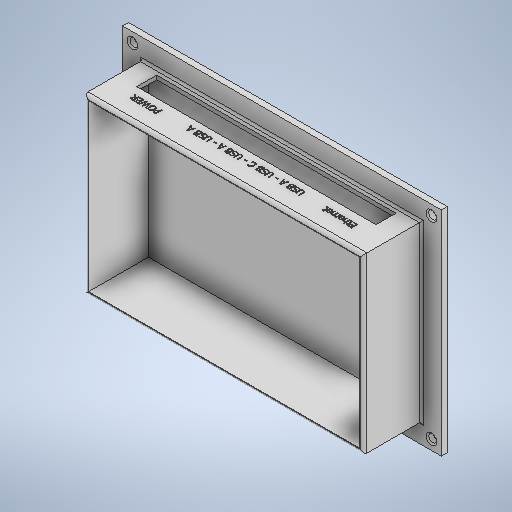
# Autodesk Inventor part: DS Holder
Saved by Autodesk Inventor 2025.1 (Build 291241000, 241)
## iProperties
Created: 2024-09-14
Part Number: DS Holder
Material: Generic
Document SubType Name: Modeling
Designer: ishaa
Density: 1 g/cm^3
Appearance: Default
Author: ishaa
## iProperties of the stored document DS Holder_3DPrint.ipt
Created: 2024-09-15
Part Number: DS Holder_3DPrint
Material: Generic
Document SubType Name: Modeling
Designer: ishaa
Density: 1 g/cm^3
Appearance: Default
Author: ishaa
Autodesk Inventor part; units mm, degrees
ref_plane "YZ Plane" through (0, 0, 0) normal (1, 0, 0) x (0, 1, 0)
ref_plane "XZ Plane" through (0, 0, 0) normal (0, 1, 0) x (-1, 0, 0)
ref_plane "XY Plane" through (0, 0, 0) normal (0, 0, 1) x (1, 0, 0)
sketch "Sketch1" plane through (0, 0, 0) normal (0, 0, 1) x (1, 0, 0)
  line L0 (-70, -43.5) -> (70, -43.5)
  line L1 (70, -43.5) -> (70, 43.5)
  line L2 (70, 43.5) -> (-70, 43.5)
  line L3 (-70, 43.5) -> (-70, -43.5)
  line L4 (-70, -43.5) -> (70, 43.5) construction
  line L5 (70, -43.5) -> (-70, 43.5) construction
  point P0 (0, 0)
  dimension "d0" = 140
  dimension "d1" = 87
  constraints: 12 end point, 2 midpoint, 2 parallel, 1 horizontal, 1 perpendicular
  measures "d0" distance of L2.end L1.end
  measures "d1" distance of L1.end L0.end
extrude "Extrusion1" add sketch "Sketch1" along normal blind 2
sketch "Sketch2" plane through (0, 0, 2) normal (0, 0, 1) x (1, 0, 0)
  line L0 (70, -43.5) -> (70, 43.5) projected
  line L1 (70, 43.5) -> (-70, 43.5) projected
  line L2 (-70, 43.5) -> (-70, -43.5) projected
  line L3 (-70, -43.5) -> (70, -43.5) projected
  line L4 (-68, 41.5) -> (68, 41.5)
  line L5 (68, 41.5) -> (68, -41.5)
  line L6 (68, -41.5) -> (-68, -41.5)
  line L7 (-68, -41.5) -> (-68, 41.5)
  point P0 (0, 0)
  dimension "d4" = 2
  constraints: 8 end point, 3 other
  measures "d4" distance between parallel lines of L1 L4
extrude "Extrusion2" add sketch "Sketch2" along normal blind 30
sketch "Sketch3" plane through (0, 0, 0) normal (0, 0, -1) x (-1, 0, 0)
  line L0 (-70, -43.5) -> (-70, 43.5) projected
  line L1 (70, -43.5) -> (-70, -43.5) projected
  line L2 (70, 43.5) -> (70, -43.5) projected
  line L3 (-70, 43.5) -> (70, 43.5) projected
  line L4 (80, -53.5) -> (-80, -53.5)
  line L5 (-80, -53.5) -> (-80, 53.5)
  line L6 (-80, 53.5) -> (80, 53.5)
  line L7 (80, 53.5) -> (80, -53.5)
  point P0 (0, 0)
  dimension "d7" = 10
  constraints: 8 end point, 3 other
  measures "d7" distance between parallel lines of L2 L7
extrude "Extrusion3" add sketch "Sketch3" against normal blind 3
sketch "Sketch4" plane through (-70, 43.5, 32) normal (0, 1, 0) x (1, 0, 0)
  line L0 (140, 29) -> (0, 29) projected
  line L1 (0, 29) -> (0, 0) projected
  line L2 (140, 0) -> (0, 0) projected
  line L3 (140, 29) -> (140, 0) projected
  line L4 (140, 0) -> (0, 29) construction
  line L5 (140, 29) -> (0, 0) construction
  line L6 (70, 0) -> (70, 29) construction
  line L7 (140, 14.5) -> (0, 14.5) construction
  line L8 (150, 29) -> (-10, 29) construction
  line L9 (70, 26.2) -> (0, 26.2) construction
  line L10 (70, 26.2) -> (140, 26.2) construction
  line L11 (130, 26.2) -> (10, 26.2)
  line L12 (10, 26.2) -> (10, 16.2)
  line L13 (10, 16.2) -> (130, 16.2)
  line L14 (130, 16.2) -> (130, 26.2)
  line L15 (130, 26.2) -> (10, 16.2) construction
  line L16 (10, 26.2) -> (130, 16.2) construction
  point P0 (70, 32)
  point P1 (70, 21.2)
  dimension "d10" = 2.8
  dimension "d11" = 5
  dimension "d12" = 120
  dimension "d13" = 10
  constraints: 24 end point, 7 midpoint, 5 point on line, 2 parallel, 2 perpendicular, 1 horizontal
  measures "d10" distance of point (70, 29) L9.start
  measures "d11" distance of L9.start point (70, 21.2)
  measures "d12" distance of L13.end L12.end
  measures "d13" distance of L12.end L11.end
extrude "Extrusion4" cut sketch "Sketch4" against normal blind 33.1625 contours L14 L13 L12 L11
sketch "Sketch5" plane through (-70, 43.5, 32) normal (0, 1, 0) x (1, 0, 0)
  line L0 (26.8965, 6.9615) -> (8.442, 6.9615) construction
  line L1 (8.442, 6.9615) -> (8.442, 14.5893) construction
  line L2 (8.442, 14.5893) -> (26.8965, 14.5893) construction
  line L3 (26.8965, 14.5893) -> (26.8965, 6.9615) construction
  line L4 (98.3767, 9.7911) -> (24.4359, 9.7911) construction
  line L5 (24.4359, 9.7911) -> (24.4359, 16.5578) construction
  line L6 (24.4359, 16.5578) -> (98.3767, 16.5578) construction
  line L7 (98.3767, 16.5578) -> (98.3767, 9.7911) construction
  line L8 (125.5663, 8.5608) -> (105.3894, 8.5608) construction
  line L9 (105.3894, 8.5608) -> (105.3894, 15.8196) construction
  line L10 (105.3894, 15.8196) -> (125.5663, 15.8196) construction
  line L11 (125.5663, 15.8196) -> (125.5663, 8.5608) construction
  line L12 (125.2575, 11.7447) -> (125.2575, 8.6967)
  line L13 (125.2575, 8.6967) -> (123.3507, 8.6967)
  line L14 (123.3507, 8.6967) -> (123.3507, 9.0573)
  line L15 (123.3507, 9.0573) -> (124.8524, 9.0573)
  line L16 (124.8524, 9.0573) -> (124.8524, 9.8922)
  line L17 (124.8524, 9.8922) -> (123.4519, 9.8922)
  line L18 (123.4519, 9.8922) -> (123.4519, 10.2528)
  line L19 (123.4519, 10.2528) -> (124.8524, 10.2528)
  line L20 (124.8524, 10.2528) -> (124.8524, 11.3841)
  line L21 (124.8524, 11.3841) -> (123.3507, 11.3841)
  line L22 (123.3507, 11.3841) -> (123.3507, 11.7447)
  line L23 (123.3507, 11.7447) -> (125.2575, 11.7447)
  spline S0 degree 2 poles (122.2441, 11.7892) (122.5578, 11.7892) (122.911, 11.431) (122.911, 11.0432) knots 0 0 0 1 2 2 2
  line L24 (122.911, 11.0432) -> (122.911, 9.7761)
  line L25 (122.911, 9.7761) -> (123.1704, 9.7761)
  line L26 (123.1704, 9.7761) -> (123.1704, 9.4575)
  line L27 (123.1704, 9.4575) -> (122.911, 9.4575)
  line L28 (122.911, 9.4575) -> (122.911, 8.8004)
  line L29 (122.911, 8.8004) -> (122.5257, 8.8004)
  line L30 (122.5257, 8.8004) -> (122.5257, 9.4575)
  line L31 (122.5257, 9.4575) -> (121.8168, 9.4575)
  line L32 (121.8168, 9.4575) -> (121.8168, 9.7761)
  line L33 (121.8168, 9.7761) -> (122.5257, 9.7761)
  line L34 (122.5257, 9.7761) -> (122.5257, 10.8654)
  spline S1 degree 2 poles (122.5257, 10.8654) (122.5257, 11.0383) (122.5133, 11.2285) (122.4713, 11.31) knots 0 0 0 1 2 2 2
  spline S2 degree 2 poles (122.4713, 11.31) (122.4368, 11.3816) (122.2812, 11.4532) (122.1478, 11.4532) knots 0 0 0 1 2 2 2
  spline S3 degree 2 poles (122.1478, 11.4532) (122.0539, 11.4532) (121.8785, 11.3964) (121.839, 11.3791) knots 0 0 0 1 2 2 2
  line L35 (121.839, 11.3791) -> (121.8168, 11.3791)
  line L36 (121.8168, 11.3791) -> (121.8168, 11.7249)
  spline S4 degree 2 poles (121.8168, 11.7249) (121.9255, 11.7546) (122.1478, 11.7892) (122.2441, 11.7892) knots 0 0 0 1 2 2 2
  line L37 (119.737, 11.7447) -> (120.1224, 11.7447)
  line L38 (120.1224, 11.7447) -> (120.1224, 10.4405)
  spline S5 degree 2 poles (120.1224, 10.4405) (120.1224, 10.2824) (120.152, 10.0107) (120.1965, 9.9292) knots 0 0 0 1 2 2 2
  spline S6 degree 2 poles (120.1965, 9.9292) (120.2434, 9.8428) (120.4114, 9.7588) (120.5546, 9.7588) knots 0 0 0 1 2 2 2
  spline S7 degree 2 poles (120.5546, 9.7588) (120.6979, 9.7588) (121.0017, 9.9119) (121.1474, 10.0354) knots 0 0 0 1 2 2 2
  line L39 (121.1474, 10.0354) -> (121.1474, 11.7447)
  line L40 (121.1474, 11.7447) -> (121.5327, 11.7447)
  line L41 (121.5327, 11.7447) -> (121.5327, 8.5608)
  line L42 (121.5327, 8.5608) -> (121.1474, 8.5608)
  line L43 (121.1474, 8.5608) -> (121.1474, 9.7119)
  spline S8 degree 2 poles (121.1474, 9.7119) (120.9745, 9.5563) (120.6411, 9.3932) (120.4533, 9.3932) knots 0 0 0 1 2 2 2
  spline S9 degree 2 poles (120.4533, 9.3932) (120.1174, 9.3932) (119.737, 9.8378) (119.737, 10.2602) knots 0 0 0 1 2 2 2
  line L44 (119.737, 10.2602) -> (119.737, 11.7447)
  spline S10 degree 2 poles (118.2032, 11.7966) (118.7515, 11.7966) (119.3542, 11.1815) (119.3542, 10.6134) knots 0 0 0 1 2 2 2
  spline S11 degree 2 poles (119.3542, 10.6134) (119.3542, 10.0552) (118.7688, 9.3932) (118.297, 9.3932) knots 0 0 0 1 2 2 2
  spline S12 degree 2 poles (118.297, 9.3932) (118.0846, 9.3932) (117.7561, 9.5167) (117.6351, 9.6477) knots 0 0 0 1 2 2 2
  spline S13 degree 2 poles (117.6351, 9.6477) (117.5116, 9.7786) (117.3806, 10.1565) (117.3806, 10.4306) knots 0 0 0 1 2 2 2
  line L45 (117.3806, 10.4306) -> (117.3806, 10.6406)
  line L46 (117.3806, 10.6406) -> (118.9639, 10.6406)
  spline S14 degree 2 poles (118.9639, 10.6406) (118.9639, 11.0383) (118.5638, 11.4606) (118.2081, 11.4606) knots 0 0 0 1 2 2 2
  spline S15 degree 2 poles (118.2081, 11.4606) (118.0821, 11.4606) (117.8376, 11.4038) (117.7388, 11.3594) knots 0 0 0 1 2 2 2
  spline S16 degree 2 poles (117.7388, 11.3594) (117.6351, 11.31) (117.4918, 11.2235) (117.4449, 11.184) knots 0 0 0 1 2 2 2
  line L47 (117.4449, 11.184) -> (117.4226, 11.184)
  line L48 (117.4226, 11.184) -> (117.4226, 11.6039)
  spline S17 degree 2 poles (117.4226, 11.6039) (117.4893, 11.6311) (117.6919, 11.7101) (117.7709, 11.7323) knots 0 0 0 1 2 2 2
  spline S18 degree 2 poles (117.7709, 11.7323) (117.8821, 11.7645) (118.0648, 11.7966) (118.2032, 11.7966) knots 0 0 0 1 2 2 2
  spline S19 degree 2 poles (117.7561, 10.3467) (117.761, 10.1911) (117.8252, 9.9638) (117.887, 9.8872) knots 0 0 0 1 2 2 2
  spline S20 degree 2 poles (117.887, 9.8872) (117.9537, 9.8008) (118.1636, 9.7094) (118.3193, 9.7094) knots 0 0 0 1 2 2 2
  spline S21 degree 2 poles (118.3193, 9.7094) (118.4724, 9.7094) (118.6873, 9.8008) (118.7762, 9.8897) knots 0 0 0 1 2 2 2
  spline S22 degree 2 poles (118.7762, 9.8897) (118.8627, 9.9811) (118.9516, 10.2009) (118.9639, 10.3467) knots 0 0 0 1 2 2 2
  line L49 (118.9639, 10.3467) -> (117.7561, 10.3467)
  line L50 (115.7776, 9.87) -> (115.7974, 9.87)
  spline S23 degree 2 poles (115.7974, 9.87) (115.8418, 9.8576) (115.9382, 9.8527) (116.0048, 9.8527) knots 0 0 0 1 2 2 2
  spline S24 degree 2 poles (116.0048, 9.8527) (116.1605, 9.8527) (116.4667, 9.9885) (116.6051, 10.1219) knots 0 0 0 1 2 2 2
  line L51 (116.6051, 10.1219) -> (116.6051, 11.7447)
  line L52 (116.6051, 11.7447) -> (116.9904, 11.7447)
  line L53 (116.9904, 11.7447) -> (116.9904, 9.4575)
  line L54 (116.9904, 9.4575) -> (116.6051, 9.4575)
  line L55 (116.6051, 9.4575) -> (116.6051, 9.7983)
  spline S25 degree 2 poles (116.6051, 9.7983) (116.3951, 9.6106) (116.0814, 9.4575) (115.9332, 9.4575) knots 0 0 0 1 2 2 2
  spline S26 degree 2 poles (115.9332, 9.4575) (115.8739, 9.4575) (115.8147, 9.4624) (115.7776, 9.4698) knots 0 0 0 1 2 2 2
  line L56 (115.7776, 9.4698) -> (115.7776, 9.87)
  line L57 (113.683, 11.7447) -> (114.0684, 11.7447)
  line L58 (114.0684, 11.7447) -> (114.0684, 10.4405)
  spline S27 degree 2 poles (114.0684, 10.4405) (114.0684, 10.2824) (114.098, 10.0107) (114.1425, 9.9292) knots 0 0 0 1 2 2 2
  spline S28 degree 2 poles (114.1425, 9.9292) (114.1894, 9.8428) (114.3573, 9.7588) (114.5006, 9.7588) knots 0 0 0 1 2 2 2
  spline S29 degree 2 poles (114.5006, 9.7588) (114.6439, 9.7588) (114.9477, 9.9119) (115.0934, 10.0354) knots 0 0 0 1 2 2 2
  line L59 (115.0934, 10.0354) -> (115.0934, 11.7447)
  line L60 (115.0934, 11.7447) -> (115.4787, 11.7447)
  line L61 (115.4787, 11.7447) -> (115.4787, 9.4575)
  line L62 (115.4787, 9.4575) -> (115.0934, 9.4575)
  line L63 (115.0934, 9.4575) -> (115.0934, 9.7119)
  spline S30 degree 2 poles (115.0934, 9.7119) (114.9205, 9.5563) (114.5871, 9.3932) (114.3993, 9.3932) knots 0 0 0 1 2 2 2
  spline S31 degree 2 poles (114.3993, 9.3932) (114.0634, 9.3932) (113.683, 9.8378) (113.683, 10.2602) knots 0 0 0 1 2 2 2
  line L64 (113.683, 10.2602) -> (113.683, 11.7447)
  spline S32 degree 2 poles (112.1492, 11.7966) (112.6975, 11.7966) (113.3002, 11.1815) (113.3002, 10.6134) knots 0 0 0 1 2 2 2
  spline S33 degree 2 poles (113.3002, 10.6134) (113.3002, 10.0552) (112.7148, 9.3932) (112.243, 9.3932) knots 0 0 0 1 2 2 2
  spline S34 degree 2 poles (112.243, 9.3932) (112.0306, 9.3932) (111.7021, 9.5167) (111.581, 9.6477) knots 0 0 0 1 2 2 2
  spline S35 degree 2 poles (111.581, 9.6477) (111.4575, 9.7786) (111.3266, 10.1565) (111.3266, 10.4306) knots 0 0 0 1 2 2 2
  line L65 (111.3266, 10.4306) -> (111.3266, 10.6406)
  line L66 (111.3266, 10.6406) -> (112.9099, 10.6406)
  spline S36 degree 2 poles (112.9099, 10.6406) (112.9099, 11.0383) (112.5098, 11.4606) (112.1541, 11.4606) knots 0 0 0 1 2 2 2
  spline S37 degree 2 poles (112.1541, 11.4606) (112.0281, 11.4606) (111.7836, 11.4038) (111.6848, 11.3594) knots 0 0 0 1 2 2 2
  spline S38 degree 2 poles (111.6848, 11.3594) (111.581, 11.31) (111.4378, 11.2235) (111.3909, 11.184) knots 0 0 0 1 2 2 2
  line L67 (111.3909, 11.184) -> (111.3686, 11.184)
  line L68 (111.3686, 11.184) -> (111.3686, 11.6039)
  spline S39 degree 2 poles (111.3686, 11.6039) (111.4353, 11.6311) (111.6379, 11.7101) (111.7169, 11.7323) knots 0 0 0 1 2 2 2
  spline S40 degree 2 poles (111.7169, 11.7323) (111.828, 11.7645) (112.0108, 11.7966) (112.1492, 11.7966) knots 0 0 0 1 2 2 2
  spline S41 degree 2 poles (111.7021, 10.3467) (111.707, 10.1911) (111.7712, 9.9638) (111.833, 9.8872) knots 0 0 0 1 2 2 2
  spline S42 degree 2 poles (111.833, 9.8872) (111.8997, 9.8008) (112.1096, 9.7094) (112.2652, 9.7094) knots 0 0 0 1 2 2 2
  spline S43 degree 2 poles (112.2652, 9.7094) (112.4184, 9.7094) (112.6333, 9.8008) (112.7222, 9.8897) knots 0 0 0 1 2 2 2
  spline S44 degree 2 poles (112.7222, 9.8897) (112.8086, 9.9811) (112.8976, 10.2009) (112.9099, 10.3467) knots 0 0 0 1 2 2 2
  line L69 (112.9099, 10.3467) -> (111.7021, 10.3467)
  spline S45 degree 2 poles (110.2448, 11.7892) (110.5585, 11.7892) (110.9117, 11.431) (110.9117, 11.0432) knots 0 0 0 1 2 2 2
  line L70 (110.9117, 11.0432) -> (110.9117, 9.7761)
  line L71 (110.9117, 9.7761) -> (111.171, 9.7761)
  line L72 (111.171, 9.7761) -> (111.171, 9.4575)
  line L73 (111.171, 9.4575) -> (110.9117, 9.4575)
  line L74 (110.9117, 9.4575) -> (110.9117, 8.8004)
  line L75 (110.9117, 8.8004) -> (110.5264, 8.8004)
  line L76 (110.5264, 8.8004) -> (110.5264, 9.4575)
  line L77 (110.5264, 9.4575) -> (109.8175, 9.4575)
  line L78 (109.8175, 9.4575) -> (109.8175, 9.7761)
  line L79 (109.8175, 9.7761) -> (110.5264, 9.7761)
  line L80 (110.5264, 9.7761) -> (110.5264, 10.8654)
  spline S46 degree 2 poles (110.5264, 10.8654) (110.5264, 11.0383) (110.514, 11.2285) (110.472, 11.31) knots 0 0 0 1 2 2 2
  spline S47 degree 2 poles (110.472, 11.31) (110.4374, 11.3816) (110.2818, 11.4532) (110.1484, 11.4532) knots 0 0 0 1 2 2 2
  spline S48 degree 2 poles (110.1484, 11.4532) (110.0546, 11.4532) (109.8792, 11.3964) (109.8397, 11.3791) knots 0 0 0 1 2 2 2
  line L81 (109.8397, 11.3791) -> (109.8175, 11.3791)
  line L82 (109.8175, 11.3791) -> (109.8175, 11.7249)
  spline S49 degree 2 poles (109.8175, 11.7249) (109.9261, 11.7546) (110.1484, 11.7892) (110.2448, 11.7892) knots 0 0 0 1 2 2 2
  spline S50 degree 2 poles (97.0034, 12.9577) (97.2726, 12.9577) (97.6728, 12.8169) (97.8136, 12.6761) knots 0 0 0 1 2 2 2
  spline S51 degree 2 poles (97.8136, 12.6761) (97.9741, 12.518) (98.105, 12.0734) (98.105, 11.7474) knots 0 0 0 1 2 2 2
  line L83 (98.105, 11.7474) -> (98.105, 9.8455)
  line L84 (98.105, 9.8455) -> (97.6999, 9.8455)
  line L85 (97.6999, 9.8455) -> (97.6999, 11.7474)
  spline S52 degree 2 poles (97.6999, 11.7474) (97.6999, 11.9598) (97.6456, 12.2463) (97.569, 12.3624) knots 0 0 0 1 2 2 2
  spline S53 degree 2 poles (97.569, 12.3624) (97.4875, 12.4859) (97.2059, 12.6119) (97.0034, 12.6119) knots 0 0 0 1 2 2 2
  spline S54 degree 2 poles (97.0034, 12.6119) (96.8132, 12.6119) (96.5168, 12.4859) (96.4353, 12.3624) knots 0 0 0 1 2 2 2
  spline S55 degree 2 poles (96.4353, 12.3624) (96.3587, 12.2463) (96.3044, 11.9623) (96.3044, 11.7573) knots 0 0 0 1 2 2 2
  line L86 (96.3044, 11.7573) -> (96.3044, 9.8455)
  line L87 (96.3044, 9.8455) -> (95.8993, 9.8455)
  line L88 (95.8993, 9.8455) -> (95.8993, 11.7474)
  spline S56 degree 2 poles (95.8993, 11.7474) (95.8993, 12.066) (96.0277, 12.5205) (96.1908, 12.6761) knots 0 0 0 1 2 2 2
  spline S57 degree 2 poles (96.1908, 12.6761) (96.3365, 12.8194) (96.7218, 12.9577) (97.0034, 12.9577) knots 0 0 0 1 2 2 2
  spline S58 degree 2 poles (94.4692, 12.9478) (94.8001, 12.9478) (95.2645, 12.8095) (95.4695, 12.7107) knots 0 0 0 1 2 2 2
  line L89 (95.4695, 12.7107) -> (95.4695, 12.2019)
  line L90 (95.4695, 12.2019) -> (95.4399, 12.2019)
  spline S59 degree 2 poles (95.4399, 12.2019) (95.2398, 12.3896) (94.7334, 12.5971) (94.4988, 12.5971) knots 0 0 0 1 2 2 2
  spline S60 degree 2 poles (94.4988, 12.5971) (94.1629, 12.5971) (93.8195, 12.318) (93.8195, 12.0883) knots 0 0 0 1 2 2 2
  spline S61 degree 2 poles (93.8195, 12.0883) (93.8195, 11.9055) (93.9998, 11.6782) (94.195, 11.6214) knots 0 0 0 1 2 2 2
  spline S62 degree 2 poles (94.195, 11.6214) (94.3358, 11.5819) (94.5704, 11.5276) (94.7458, 11.4831) knots 0 0 0 1 2 2 2
  spline S63 degree 2 poles (94.7458, 11.4831) (94.9039, 11.4411) (95.1533, 11.3151) (95.2497, 11.2139) knots 0 0 0 1 2 2 2
  spline S64 degree 2 poles (95.2497, 11.2139) (95.3435, 11.1126) (95.4473, 10.8409) (95.4473, 10.6631) knots 0 0 0 1 2 2 2
  spline S65 degree 2 poles (95.4473, 10.6631) (95.4473, 10.2926) (94.8693, 9.7911) (94.4222, 9.7911) knots 0 0 0 1 2 2 2
  spline S66 degree 2 poles (94.4222, 9.7911) (94.1653, 9.7911) (93.7109, 9.8924) (93.5157, 9.9887) knots 0 0 0 1 2 2 2
  line L91 (93.5157, 9.9887) -> (93.5157, 10.4729)
  line L92 (93.5157, 10.4729) -> (93.5454, 10.4729)
  spline S67 degree 2 poles (93.5454, 10.4729) (93.6911, 10.3395) (94.1456, 10.1419) (94.3951, 10.1419) knots 0 0 0 1 2 2 2
  spline S68 degree 2 poles (94.3951, 10.1419) (94.6766, 10.1419) (95.0249, 10.4062) (95.0249, 10.6211) knots 0 0 0 1 2 2 2
  spline S69 degree 2 poles (95.0249, 10.6211) (95.0249, 10.8137) (94.8199, 11.0434) (94.6272, 11.0953) knots 0 0 0 1 2 2 2
  spline S70 degree 2 poles (94.6272, 11.0953) (94.4988, 11.1299) (94.1258, 11.2188) (94.0023, 11.2559) knots 0 0 0 1 2 2 2
  spline S71 degree 2 poles (94.0023, 11.2559) (93.6886, 11.3522) (93.3972, 11.74) (93.3972, 12.024) knots 0 0 0 1 2 2 2
  spline S72 degree 2 poles (93.3972, 12.024) (93.3972, 12.2044) (93.5429, 12.5502) (93.6738, 12.6712) knots 0 0 0 1 2 2 2
  spline S73 degree 2 poles (93.6738, 12.6712) (93.8195, 12.8046) (94.19, 12.9478) (94.4692, 12.9478) knots 0 0 0 1 2 2 2
  spline S74 degree 2 poles (90.9173, 11.9573) (90.9173, 12.1846) (91.0902, 12.5329) (91.2334, 12.6465) knots 0 0 0 1 2 2 2
  spline S75 degree 2 poles (91.2334, 12.6465) (91.4063, 12.7799) (91.7991, 12.8935) (92.1103, 12.8935) knots 0 0 0 1 2 2 2
  line L93 (92.1103, 12.8935) -> (92.9847, 12.8935)
  line L94 (92.9847, 12.8935) -> (92.9847, 9.8455)
  line L95 (92.9847, 9.8455) -> (92.177, 9.8455)
  spline S76 degree 2 poles (92.177, 9.8455) (91.8509, 9.8455) (91.5249, 9.8875) (91.3767, 9.969) knots 0 0 0 1 2 2 2
  spline S77 degree 2 poles (91.3767, 9.969) (91.2112, 10.0554) (91.0605, 10.3395) (91.0605, 10.5321) knots 0 0 0 1 2 2 2
  spline S78 degree 2 poles (91.0605, 10.5321) (91.0605, 10.747) (91.2878, 11.0879) (91.4878, 11.1842) knots 0 0 0 1 2 2 2
  line L96 (91.4878, 11.1842) -> (91.4878, 11.1991)
  spline S79 degree 2 poles (91.4878, 11.1991) (91.2161, 11.2732) (90.9173, 11.6659) (90.9173, 11.9573) knots 0 0 0 1 2 2 2
  spline S80 degree 2 poles (91.3396, 11.9746) (91.3396, 11.8017) (91.4384, 11.5794) (91.5866, 11.5004) knots 0 0 0 1 2 2 2
  spline S81 degree 2 poles (91.5866, 11.5004) (91.683, 11.451) (91.9102, 11.4214) (92.1202, 11.4214) knots 0 0 0 1 2 2 2
  line L97 (92.1202, 11.4214) -> (92.5796, 11.4214)
  line L98 (92.5796, 11.4214) -> (92.5796, 12.5477)
  line L99 (92.5796, 12.5477) -> (92.2511, 12.5477)
  spline S82 degree 2 poles (92.2511, 12.5477) (91.9843, 12.5477) (91.678, 12.4983) (91.5595, 12.4192) knots 0 0 0 1 2 2 2
  spline S83 degree 2 poles (91.5595, 12.4192) (91.4459, 12.3377) (91.3396, 12.1352) (91.3396, 11.9746) knots 0 0 0 1 2 2 2
  spline S84 degree 2 poles (91.4829, 10.589) (91.4829, 10.4803) (91.557, 10.3173) (91.6385, 10.2703) knots 0 0 0 1 2 2 2
  spline S85 degree 2 poles (91.6385, 10.2703) (91.7373, 10.216) (91.9769, 10.1913) (92.1918, 10.1913) knots 0 0 0 1 2 2 2
  line L100 (92.1918, 10.1913) -> (92.5796, 10.1913)
  line L101 (92.5796, 10.1913) -> (92.5796, 11.083)
  line L102 (92.5796, 11.083) -> (92.1202, 11.083)
  spline S86 degree 2 poles (92.1202, 11.083) (91.93, 11.083) (91.7497, 11.0434) (91.6533, 10.9817) knots 0 0 0 1 2 2 2
  spline S87 degree 2 poles (91.6533, 10.9817) (91.5595, 10.9224) (91.4829, 10.7322) (91.4829, 10.589) knots 0 0 0 1 2 2 2
  line L103 (89.5341, 12.8935) -> (88.5065, 9.8455)
  line L104 (88.5065, 9.8455) -> (88.0076, 9.8455)
  line L105 (88.0076, 9.8455) -> (86.9801, 12.8935)
  line L106 (86.9801, 12.8935) -> (87.4074, 12.8935)
  line L107 (87.4074, 12.8935) -> (87.684, 12.0413)
  line L108 (87.684, 12.0413) -> (88.8474, 12.0413)
  line L109 (88.8474, 12.0413) -> (89.124, 12.8935)
  line L110 (89.124, 12.8935) -> (89.5341, 12.8935)
  line L111 (87.7952, 11.6955) -> (88.2669, 10.2604)
  line L112 (88.2669, 10.2604) -> (88.7362, 11.6955)
  line L113 (88.7362, 11.6955) -> (87.7952, 11.6955)
  line L114 (84.352, 11.7449) -> (85.5055, 11.7449)
  line L115 (85.5055, 11.7449) -> (85.5055, 11.3744)
  line L116 (85.5055, 11.3744) -> (84.352, 11.3744)
  line L117 (84.352, 11.3744) -> (84.352, 11.7449)
  spline S88 degree 2 poles (81.4867, 12.9577) (81.756, 12.9577) (82.1561, 12.8169) (82.2969, 12.6761) knots 0 0 0 1 2 2 2
  spline S89 degree 2 poles (82.2969, 12.6761) (82.4575, 12.518) (82.5884, 12.0734) (82.5884, 11.7474) knots 0 0 0 1 2 2 2
  line L118 (82.5884, 11.7474) -> (82.5884, 9.8455)
  line L119 (82.5884, 9.8455) -> (82.1833, 9.8455)
  line L120 (82.1833, 9.8455) -> (82.1833, 11.7474)
  spline S90 degree 2 poles (82.1833, 11.7474) (82.1833, 11.9598) (82.129, 12.2463) (82.0524, 12.3624) knots 0 0 0 1 2 2 2
  spline S91 degree 2 poles (82.0524, 12.3624) (81.9709, 12.4859) (81.6893, 12.6119) (81.4867, 12.6119) knots 0 0 0 1 2 2 2
  spline S92 degree 2 poles (81.4867, 12.6119) (81.2966, 12.6119) (81.0002, 12.4859) (80.9186, 12.3624) knots 0 0 0 1 2 2 2
  spline S93 degree 2 poles (80.9186, 12.3624) (80.8421, 12.2463) (80.7877, 11.9623) (80.7877, 11.7573) knots 0 0 0 1 2 2 2
  line L121 (80.7877, 11.7573) -> (80.7877, 9.8455)
  line L122 (80.7877, 9.8455) -> (80.3826, 9.8455)
  line L123 (80.3826, 9.8455) -> (80.3826, 11.7474)
  spline S94 degree 2 poles (80.3826, 11.7474) (80.3826, 12.066) (80.5111, 12.5205) (80.6741, 12.6761) knots 0 0 0 1 2 2 2
  spline S95 degree 2 poles (80.6741, 12.6761) (80.8198, 12.8194) (81.2052, 12.9577) (81.4867, 12.9577) knots 0 0 0 1 2 2 2
  spline S96 degree 2 poles (78.9525, 12.9478) (79.2835, 12.9478) (79.7479, 12.8095) (79.9529, 12.7107) knots 0 0 0 1 2 2 2
  line L124 (79.9529, 12.7107) -> (79.9529, 12.2019)
  line L125 (79.9529, 12.2019) -> (79.9232, 12.2019)
  spline S97 degree 2 poles (79.9232, 12.2019) (79.7232, 12.3896) (79.2168, 12.5971) (78.9821, 12.5971) knots 0 0 0 1 2 2 2
  spline S98 degree 2 poles (78.9821, 12.5971) (78.6462, 12.5971) (78.3029, 12.318) (78.3029, 12.0883) knots 0 0 0 1 2 2 2
  spline S99 degree 2 poles (78.3029, 12.0883) (78.3029, 11.9055) (78.4832, 11.6782) (78.6783, 11.6214) knots 0 0 0 1 2 2 2
  spline S100 degree 2 poles (78.6783, 11.6214) (78.8191, 11.5819) (79.0538, 11.5276) (79.2292, 11.4831) knots 0 0 0 1 2 2 2
  spline S101 degree 2 poles (79.2292, 11.4831) (79.3872, 11.4411) (79.6367, 11.3151) (79.733, 11.2139) knots 0 0 0 1 2 2 2
  spline S102 degree 2 poles (79.733, 11.2139) (79.8269, 11.1126) (79.9306, 10.8409) (79.9306, 10.6631) knots 0 0 0 1 2 2 2
  spline S103 degree 2 poles (79.9306, 10.6631) (79.9306, 10.2926) (79.3527, 9.7911) (78.9056, 9.7911) knots 0 0 0 1 2 2 2
  spline S104 degree 2 poles (78.9056, 9.7911) (78.6487, 9.7911) (78.1942, 9.8924) (77.9991, 9.9887) knots 0 0 0 1 2 2 2
  line L126 (77.9991, 9.9887) -> (77.9991, 10.4729)
  line L127 (77.9991, 10.4729) -> (78.0287, 10.4729)
  spline S105 degree 2 poles (78.0287, 10.4729) (78.1745, 10.3395) (78.6289, 10.1419) (78.8784, 10.1419) knots 0 0 0 1 2 2 2
  spline S106 degree 2 poles (78.8784, 10.1419) (79.16, 10.1419) (79.5083, 10.4062) (79.5083, 10.6211) knots 0 0 0 1 2 2 2
  spline S107 degree 2 poles (79.5083, 10.6211) (79.5083, 10.8137) (79.3033, 11.0434) (79.1106, 11.0953) knots 0 0 0 1 2 2 2
  spline S108 degree 2 poles (79.1106, 11.0953) (78.9821, 11.1299) (78.6092, 11.2188) (78.4857, 11.2559) knots 0 0 0 1 2 2 2
  spline S109 degree 2 poles (78.4857, 11.2559) (78.172, 11.3522) (77.8805, 11.74) (77.8805, 12.024) knots 0 0 0 1 2 2 2
  spline S110 degree 2 poles (77.8805, 12.024) (77.8805, 12.2044) (78.0263, 12.5502) (78.1572, 12.6712) knots 0 0 0 1 2 2 2
  spline S111 degree 2 poles (78.1572, 12.6712) (78.3029, 12.8046) (78.6734, 12.9478) (78.9525, 12.9478) knots 0 0 0 1 2 2 2
  spline S112 degree 2 poles (75.4006, 11.9573) (75.4006, 12.1846) (75.5735, 12.5329) (75.7168, 12.6465) knots 0 0 0 1 2 2 2
  spline S113 degree 2 poles (75.7168, 12.6465) (75.8897, 12.7799) (76.2824, 12.8935) (76.5936, 12.8935) knots 0 0 0 1 2 2 2
  line L128 (76.5936, 12.8935) -> (77.468, 12.8935)
  line L129 (77.468, 12.8935) -> (77.468, 9.8455)
  line L130 (77.468, 9.8455) -> (76.6603, 9.8455)
  spline S114 degree 2 poles (76.6603, 9.8455) (76.3343, 9.8455) (76.0082, 9.8875) (75.86, 9.969) knots 0 0 0 1 2 2 2
  spline S115 degree 2 poles (75.86, 9.969) (75.6946, 10.0554) (75.5439, 10.3395) (75.5439, 10.5321) knots 0 0 0 1 2 2 2
  spline S116 degree 2 poles (75.5439, 10.5321) (75.5439, 10.747) (75.7711, 11.0879) (75.9712, 11.1842) knots 0 0 0 1 2 2 2
  line L131 (75.9712, 11.1842) -> (75.9712, 11.1991)
  spline S117 degree 2 poles (75.9712, 11.1991) (75.6995, 11.2732) (75.4006, 11.6659) (75.4006, 11.9573) knots 0 0 0 1 2 2 2
  spline S118 degree 2 poles (75.823, 11.9746) (75.823, 11.8017) (75.9218, 11.5794) (76.07, 11.5004) knots 0 0 0 1 2 2 2
  spline S119 degree 2 poles (76.07, 11.5004) (76.1663, 11.451) (76.3936, 11.4214) (76.6035, 11.4214) knots 0 0 0 1 2 2 2
  line L132 (76.6035, 11.4214) -> (77.0629, 11.4214)
  line L133 (77.0629, 11.4214) -> (77.0629, 12.5477)
  line L134 (77.0629, 12.5477) -> (76.7344, 12.5477)
  spline S120 degree 2 poles (76.7344, 12.5477) (76.4677, 12.5477) (76.1614, 12.4983) (76.0428, 12.4192) knots 0 0 0 1 2 2 2
  spline S121 degree 2 poles (76.0428, 12.4192) (75.9292, 12.3377) (75.823, 12.1352) (75.823, 11.9746) knots 0 0 0 1 2 2 2
  spline S122 degree 2 poles (75.9663, 10.589) (75.9663, 10.4803) (76.0404, 10.3173) (76.1219, 10.2703) knots 0 0 0 1 2 2 2
  spline S123 degree 2 poles (76.1219, 10.2703) (76.2207, 10.216) (76.4603, 10.1913) (76.6752, 10.1913) knots 0 0 0 1 2 2 2
  line L135 (76.6752, 10.1913) -> (77.0629, 10.1913)
  line L136 (77.0629, 10.1913) -> (77.0629, 11.083)
  line L137 (77.0629, 11.083) -> (76.6035, 11.083)
  spline S124 degree 2 poles (76.6035, 11.083) (76.4133, 11.083) (76.233, 11.0434) (76.1367, 10.9817) knots 0 0 0 1 2 2 2
  spline S125 degree 2 poles (76.1367, 10.9817) (76.0428, 10.9224) (75.9663, 10.7322) (75.9663, 10.589) knots 0 0 0 1 2 2 2
  spline S126 degree 2 poles (72.4984, 12.9478) (72.7948, 12.9478) (73.2962, 12.7478) (73.479, 12.5477) knots 0 0 0 1 2 2 2
  spline S127 degree 2 poles (73.479, 12.5477) (73.6617, 12.3501) (73.8618, 11.7573) (73.8618, 11.372) knots 0 0 0 1 2 2 2
  spline S128 degree 2 poles (73.8618, 11.372) (73.8618, 10.9891) (73.6667, 10.421) (73.4814, 10.211) knots 0 0 0 1 2 2 2
  spline S129 degree 2 poles (73.4814, 10.211) (73.2986, 10.006) (72.7997, 9.7911) (72.4909, 9.7911) knots 0 0 0 1 2 2 2
  spline S130 degree 2 poles (72.4909, 9.7911) (72.3378, 9.7911) (72.0686, 9.8356) (71.955, 9.8702) knots 0 0 0 1 2 2 2
  spline S131 degree 2 poles (71.955, 9.8702) (71.8562, 9.9023) (71.6511, 9.9937) (71.5499, 10.048) knots 0 0 0 1 2 2 2
  line L138 (71.5499, 10.048) -> (71.5499, 10.5371)
  line L139 (71.5499, 10.5371) -> (71.582, 10.5371)
  spline S132 degree 2 poles (71.582, 10.5371) (71.6363, 10.4877) (71.8043, 10.3494) (71.9253, 10.2827) knots 0 0 0 1 2 2 2
  spline S133 degree 2 poles (71.9253, 10.2827) (72.0414, 10.2185) (72.3156, 10.1369) (72.4934, 10.1369) knots 0 0 0 1 2 2 2
  spline S134 degree 2 poles (72.4934, 10.1369) (72.6885, 10.1369) (73.0368, 10.2975) (73.1677, 10.4506) knots 0 0 0 1 2 2 2
  spline S135 degree 2 poles (73.1677, 10.4506) (73.2962, 10.6062) (73.4394, 11.078) (73.4394, 11.372) knots 0 0 0 1 2 2 2
  spline S136 degree 2 poles (73.4394, 11.372) (73.4394, 11.6856) (73.2888, 12.1377) (73.1579, 12.2933) knots 0 0 0 1 2 2 2
  spline S137 degree 2 poles (73.1579, 12.2933) (73.0294, 12.4439) (72.6861, 12.5971) (72.4934, 12.5971) knots 0 0 0 1 2 2 2
  spline S138 degree 2 poles (72.4934, 12.5971) (72.318, 12.5971) (72.0192, 12.5106) (71.9031, 12.4464) knots 0 0 0 1 2 2 2
  spline S139 degree 2 poles (71.9031, 12.4464) (71.7919, 12.3822) (71.6264, 12.2488) (71.5795, 12.2019) knots 0 0 0 1 2 2 2
  line L140 (71.5795, 12.2019) -> (71.5499, 12.2019)
  line L141 (71.5499, 12.2019) -> (71.5499, 12.686)
  spline S140 degree 2 poles (71.5499, 12.686) (71.6511, 12.7329) (71.829, 12.8194) (71.955, 12.8589) knots 0 0 0 1 2 2 2
  spline S141 degree 2 poles (71.955, 12.8589) (72.0883, 12.9034) (72.3156, 12.9478) (72.4984, 12.9478) knots 0 0 0 1 2 2 2
  line L142 (68.8329, 11.7449) -> (69.9864, 11.7449)
  line L143 (69.9864, 11.7449) -> (69.9864, 11.3744)
  line L144 (69.9864, 11.3744) -> (68.8329, 11.3744)
  line L145 (68.8329, 11.3744) -> (68.8329, 11.7449)
  spline S142 degree 2 poles (65.9676, 12.9577) (66.2369, 12.9577) (66.637, 12.8169) (66.7778, 12.6761) knots 0 0 0 1 2 2 2
  spline S143 degree 2 poles (66.7778, 12.6761) (66.9384, 12.518) (67.0693, 12.0734) (67.0693, 11.7474) knots 0 0 0 1 2 2 2
  line L146 (67.0693, 11.7474) -> (67.0693, 9.8455)
  line L147 (67.0693, 9.8455) -> (66.6642, 9.8455)
  line L148 (66.6642, 9.8455) -> (66.6642, 11.7474)
  spline S144 degree 2 poles (66.6642, 11.7474) (66.6642, 11.9598) (66.6098, 12.2463) (66.5333, 12.3624) knots 0 0 0 1 2 2 2
  spline S145 degree 2 poles (66.5333, 12.3624) (66.4518, 12.4859) (66.1702, 12.6119) (65.9676, 12.6119) knots 0 0 0 1 2 2 2
  spline S146 degree 2 poles (65.9676, 12.6119) (65.7774, 12.6119) (65.481, 12.4859) (65.3995, 12.3624) knots 0 0 0 1 2 2 2
  spline S147 degree 2 poles (65.3995, 12.3624) (65.323, 12.2463) (65.2686, 11.9623) (65.2686, 11.7573) knots 0 0 0 1 2 2 2
  line L149 (65.2686, 11.7573) -> (65.2686, 9.8455)
  line L150 (65.2686, 9.8455) -> (64.8635, 9.8455)
  line L151 (64.8635, 9.8455) -> (64.8635, 11.7474)
  spline S148 degree 2 poles (64.8635, 11.7474) (64.8635, 12.066) (64.992, 12.5205) (65.155, 12.6761) knots 0 0 0 1 2 2 2
  spline S149 degree 2 poles (65.155, 12.6761) (65.3007, 12.8194) (65.6861, 12.9577) (65.9676, 12.9577) knots 0 0 0 1 2 2 2
  spline S150 degree 2 poles (63.4334, 12.9478) (63.7644, 12.9478) (64.2287, 12.8095) (64.4338, 12.7107) knots 0 0 0 1 2 2 2
  line L152 (64.4338, 12.7107) -> (64.4338, 12.2019)
  line L153 (64.4338, 12.2019) -> (64.4041, 12.2019)
  spline S151 degree 2 poles (64.4041, 12.2019) (64.204, 12.3896) (63.6977, 12.5971) (63.463, 12.5971) knots 0 0 0 1 2 2 2
  spline S152 degree 2 poles (63.463, 12.5971) (63.1271, 12.5971) (62.7838, 12.318) (62.7838, 12.0883) knots 0 0 0 1 2 2 2
  spline S153 degree 2 poles (62.7838, 12.0883) (62.7838, 11.9055) (62.9641, 11.6782) (63.1592, 11.6214) knots 0 0 0 1 2 2 2
  spline S154 degree 2 poles (63.1592, 11.6214) (63.3, 11.5819) (63.5347, 11.5276) (63.71, 11.4831) knots 0 0 0 1 2 2 2
  spline S155 degree 2 poles (63.71, 11.4831) (63.8681, 11.4411) (64.1176, 11.3151) (64.2139, 11.2139) knots 0 0 0 1 2 2 2
  spline S156 degree 2 poles (64.2139, 11.2139) (64.3078, 11.1126) (64.4115, 10.8409) (64.4115, 10.6631) knots 0 0 0 1 2 2 2
  spline S157 degree 2 poles (64.4115, 10.6631) (64.4115, 10.2926) (63.8335, 9.7911) (63.3865, 9.7911) knots 0 0 0 1 2 2 2
  spline S158 degree 2 poles (63.3865, 9.7911) (63.1296, 9.7911) (62.6751, 9.8924) (62.48, 9.9887) knots 0 0 0 1 2 2 2
  line L154 (62.48, 9.9887) -> (62.48, 10.4729)
  line L155 (62.48, 10.4729) -> (62.5096, 10.4729)
  spline S159 degree 2 poles (62.5096, 10.4729) (62.6553, 10.3395) (63.1098, 10.1419) (63.3593, 10.1419) knots 0 0 0 1 2 2 2
  spline S160 degree 2 poles (63.3593, 10.1419) (63.6409, 10.1419) (63.9892, 10.4062) (63.9892, 10.6211) knots 0 0 0 1 2 2 2
  spline S161 degree 2 poles (63.9892, 10.6211) (63.9892, 10.8137) (63.7841, 11.0434) (63.5915, 11.0953) knots 0 0 0 1 2 2 2
  spline S162 degree 2 poles (63.5915, 11.0953) (63.463, 11.1299) (63.0901, 11.2188) (62.9666, 11.2559) knots 0 0 0 1 2 2 2
  spline S163 degree 2 poles (62.9666, 11.2559) (62.6529, 11.3522) (62.3614, 11.74) (62.3614, 12.024) knots 0 0 0 1 2 2 2
  spline S164 degree 2 poles (62.3614, 12.024) (62.3614, 12.2044) (62.5071, 12.5502) (62.6381, 12.6712) knots 0 0 0 1 2 2 2
  spline S165 degree 2 poles (62.6381, 12.6712) (62.7838, 12.8046) (63.1543, 12.9478) (63.4334, 12.9478) knots 0 0 0 1 2 2 2
  spline S166 degree 2 poles (59.8815, 11.9573) (59.8815, 12.1846) (60.0544, 12.5329) (60.1977, 12.6465) knots 0 0 0 1 2 2 2
  spline S167 degree 2 poles (60.1977, 12.6465) (60.3706, 12.7799) (60.7633, 12.8935) (61.0745, 12.8935) knots 0 0 0 1 2 2 2
  line L156 (61.0745, 12.8935) -> (61.9489, 12.8935)
  line L157 (61.9489, 12.8935) -> (61.9489, 9.8455)
  line L158 (61.9489, 9.8455) -> (61.1412, 9.8455)
  spline S168 degree 2 poles (61.1412, 9.8455) (60.8152, 9.8455) (60.4891, 9.8875) (60.3409, 9.969) knots 0 0 0 1 2 2 2
  spline S169 degree 2 poles (60.3409, 9.969) (60.1754, 10.0554) (60.0248, 10.3395) (60.0248, 10.5321) knots 0 0 0 1 2 2 2
  spline S170 degree 2 poles (60.0248, 10.5321) (60.0248, 10.747) (60.252, 11.0879) (60.4521, 11.1842) knots 0 0 0 1 2 2 2
  line L159 (60.4521, 11.1842) -> (60.4521, 11.1991)
  spline S171 degree 2 poles (60.4521, 11.1991) (60.1804, 11.2732) (59.8815, 11.6659) (59.8815, 11.9573) knots 0 0 0 1 2 2 2
  spline S172 degree 2 poles (60.3039, 11.9746) (60.3039, 11.8017) (60.4027, 11.5794) (60.5509, 11.5004) knots 0 0 0 1 2 2 2
  spline S173 degree 2 poles (60.5509, 11.5004) (60.6472, 11.451) (60.8745, 11.4214) (61.0844, 11.4214) knots 0 0 0 1 2 2 2
  line L160 (61.0844, 11.4214) -> (61.5438, 11.4214)
  line L161 (61.5438, 11.4214) -> (61.5438, 12.5477)
  line L162 (61.5438, 12.5477) -> (61.2153, 12.5477)
  spline S174 degree 2 poles (61.2153, 12.5477) (60.9486, 12.5477) (60.6423, 12.4983) (60.5237, 12.4192) knots 0 0 0 1 2 2 2
  spline S175 degree 2 poles (60.5237, 12.4192) (60.4101, 12.3377) (60.3039, 12.1352) (60.3039, 11.9746) knots 0 0 0 1 2 2 2
  spline S176 degree 2 poles (60.4471, 10.589) (60.4471, 10.4803) (60.5212, 10.3173) (60.6028, 10.2703) knots 0 0 0 1 2 2 2
  spline S177 degree 2 poles (60.6028, 10.2703) (60.7016, 10.216) (60.9412, 10.1913) (61.156, 10.1913) knots 0 0 0 1 2 2 2
  line L163 (61.156, 10.1913) -> (61.5438, 10.1913)
  line L164 (61.5438, 10.1913) -> (61.5438, 11.083)
  line L165 (61.5438, 11.083) -> (61.0844, 11.083)
  spline S178 degree 2 poles (61.0844, 11.083) (60.8942, 11.083) (60.7139, 11.0434) (60.6176, 10.9817) knots 0 0 0 1 2 2 2
  spline S179 degree 2 poles (60.6176, 10.9817) (60.5237, 10.9224) (60.4471, 10.7322) (60.4471, 10.589) knots 0 0 0 1 2 2 2
  line L166 (58.4983, 12.8935) -> (57.4708, 9.8455)
  line L167 (57.4708, 9.8455) -> (56.9718, 9.8455)
  line L168 (56.9718, 9.8455) -> (55.9443, 12.8935)
  line L169 (55.9443, 12.8935) -> (56.3716, 12.8935)
  line L170 (56.3716, 12.8935) -> (56.6483, 12.0413)
  line L171 (56.6483, 12.0413) -> (57.8116, 12.0413)
  line L172 (57.8116, 12.0413) -> (58.0883, 12.8935)
  line L173 (58.0883, 12.8935) -> (58.4983, 12.8935)
  line L174 (56.7594, 11.6955) -> (57.2312, 10.2604)
  line L175 (57.2312, 10.2604) -> (57.7005, 11.6955)
  line L176 (57.7005, 11.6955) -> (56.7594, 11.6955)
  line L177 (53.3162, 11.7449) -> (54.4697, 11.7449)
  line L178 (54.4697, 11.7449) -> (54.4697, 11.3744)
  line L179 (54.4697, 11.3744) -> (53.3162, 11.3744)
  line L180 (53.3162, 11.3744) -> (53.3162, 11.7449)
  spline S180 degree 2 poles (50.451, 12.9577) (50.7202, 12.9577) (51.1204, 12.8169) (51.2612, 12.6761) knots 0 0 0 1 2 2 2
  spline S181 degree 2 poles (51.2612, 12.6761) (51.4217, 12.518) (51.5526, 12.0734) (51.5526, 11.7474) knots 0 0 0 1 2 2 2
  line L181 (51.5526, 11.7474) -> (51.5526, 9.8455)
  line L182 (51.5526, 9.8455) -> (51.1475, 9.8455)
  line L183 (51.1475, 9.8455) -> (51.1475, 11.7474)
  spline S182 degree 2 poles (51.1475, 11.7474) (51.1475, 11.9598) (51.0932, 12.2463) (51.0166, 12.3624) knots 0 0 0 1 2 2 2
  spline S183 degree 2 poles (51.0166, 12.3624) (50.9351, 12.4859) (50.6535, 12.6119) (50.451, 12.6119) knots 0 0 0 1 2 2 2
  spline S184 degree 2 poles (50.451, 12.6119) (50.2608, 12.6119) (49.9644, 12.4859) (49.8829, 12.3624) knots 0 0 0 1 2 2 2
  spline S185 degree 2 poles (49.8829, 12.3624) (49.8063, 12.2463) (49.752, 11.9623) (49.752, 11.7573) knots 0 0 0 1 2 2 2
  line L184 (49.752, 11.7573) -> (49.752, 9.8455)
  line L185 (49.752, 9.8455) -> (49.3469, 9.8455)
  line L186 (49.3469, 9.8455) -> (49.3469, 11.7474)
  spline S186 degree 2 poles (49.3469, 11.7474) (49.3469, 12.066) (49.4753, 12.5205) (49.6384, 12.6761) knots 0 0 0 1 2 2 2
  spline S187 degree 2 poles (49.6384, 12.6761) (49.7841, 12.8194) (50.1694, 12.9577) (50.451, 12.9577) knots 0 0 0 1 2 2 2
  spline S188 degree 2 poles (47.9168, 12.9478) (48.2477, 12.9478) (48.7121, 12.8095) (48.9171, 12.7107) knots 0 0 0 1 2 2 2
  line L187 (48.9171, 12.7107) -> (48.9171, 12.2019)
  line L188 (48.9171, 12.2019) -> (48.8875, 12.2019)
  spline S189 degree 2 poles (48.8875, 12.2019) (48.6874, 12.3896) (48.181, 12.5971) (47.9464, 12.5971) knots 0 0 0 1 2 2 2
  spline S190 degree 2 poles (47.9464, 12.5971) (47.6105, 12.5971) (47.2671, 12.318) (47.2671, 12.0883) knots 0 0 0 1 2 2 2
  spline S191 degree 2 poles (47.2671, 12.0883) (47.2671, 11.9055) (47.4475, 11.6782) (47.6426, 11.6214) knots 0 0 0 1 2 2 2
  spline S192 degree 2 poles (47.6426, 11.6214) (47.7834, 11.5819) (48.018, 11.5276) (48.1934, 11.4831) knots 0 0 0 1 2 2 2
  spline S193 degree 2 poles (48.1934, 11.4831) (48.3515, 11.4411) (48.6009, 11.3151) (48.6973, 11.2139) knots 0 0 0 1 2 2 2
  spline S194 degree 2 poles (48.6973, 11.2139) (48.7911, 11.1126) (48.8949, 10.8409) (48.8949, 10.6631) knots 0 0 0 1 2 2 2
  spline S195 degree 2 poles (48.8949, 10.6631) (48.8949, 10.2926) (48.3169, 9.7911) (47.8698, 9.7911) knots 0 0 0 1 2 2 2
  spline S196 degree 2 poles (47.8698, 9.7911) (47.6129, 9.7911) (47.1585, 9.8924) (46.9633, 9.9887) knots 0 0 0 1 2 2 2
  line L189 (46.9633, 9.9887) -> (46.9633, 10.4729)
  line L190 (46.9633, 10.4729) -> (46.993, 10.4729)
  spline S197 degree 2 poles (46.993, 10.4729) (47.1387, 10.3395) (47.5932, 10.1419) (47.8427, 10.1419) knots 0 0 0 1 2 2 2
  spline S198 degree 2 poles (47.8427, 10.1419) (48.1242, 10.1419) (48.4725, 10.4062) (48.4725, 10.6211) knots 0 0 0 1 2 2 2
  spline S199 degree 2 poles (48.4725, 10.6211) (48.4725, 10.8137) (48.2675, 11.0434) (48.0748, 11.0953) knots 0 0 0 1 2 2 2
  spline S200 degree 2 poles (48.0748, 11.0953) (47.9464, 11.1299) (47.5734, 11.2188) (47.4499, 11.2559) knots 0 0 0 1 2 2 2
  spline S201 degree 2 poles (47.4499, 11.2559) (47.1362, 11.3522) (46.8448, 11.74) (46.8448, 12.024) knots 0 0 0 1 2 2 2
  spline S202 degree 2 poles (46.8448, 12.024) (46.8448, 12.2044) (46.9905, 12.5502) (47.1214, 12.6712) knots 0 0 0 1 2 2 2
  spline S203 degree 2 poles (47.1214, 12.6712) (47.2671, 12.8046) (47.6376, 12.9478) (47.9168, 12.9478) knots 0 0 0 1 2 2 2
  spline S204 degree 2 poles (44.3649, 11.9573) (44.3649, 12.1846) (44.5378, 12.5329) (44.681, 12.6465) knots 0 0 0 1 2 2 2
  spline S205 degree 2 poles (44.681, 12.6465) (44.8539, 12.7799) (45.2467, 12.8935) (45.5579, 12.8935) knots 0 0 0 1 2 2 2
  line L191 (45.5579, 12.8935) -> (46.4323, 12.8935)
  line L192 (46.4323, 12.8935) -> (46.4323, 9.8455)
  line L193 (46.4323, 9.8455) -> (45.6246, 9.8455)
  spline S206 degree 2 poles (45.6246, 9.8455) (45.2985, 9.8455) (44.9725, 9.8875) (44.8243, 9.969) knots 0 0 0 1 2 2 2
  spline S207 degree 2 poles (44.8243, 9.969) (44.6588, 10.0554) (44.5081, 10.3395) (44.5081, 10.5321) knots 0 0 0 1 2 2 2
  spline S208 degree 2 poles (44.5081, 10.5321) (44.5081, 10.747) (44.7354, 11.0879) (44.9354, 11.1842) knots 0 0 0 1 2 2 2
  line L194 (44.9354, 11.1842) -> (44.9354, 11.1991)
  spline S209 degree 2 poles (44.9354, 11.1991) (44.6637, 11.2732) (44.3649, 11.6659) (44.3649, 11.9573) knots 0 0 0 1 2 2 2
  spline S210 degree 2 poles (44.7872, 11.9746) (44.7872, 11.8017) (44.886, 11.5794) (45.0342, 11.5004) knots 0 0 0 1 2 2 2
  spline S211 degree 2 poles (45.0342, 11.5004) (45.1306, 11.451) (45.3578, 11.4214) (45.5678, 11.4214) knots 0 0 0 1 2 2 2
  line L195 (45.5678, 11.4214) -> (46.0272, 11.4214)
  line L196 (46.0272, 11.4214) -> (46.0272, 12.5477)
  line L197 (46.0272, 12.5477) -> (45.6987, 12.5477)
  spline S212 degree 2 poles (45.6987, 12.5477) (45.4319, 12.5477) (45.1256, 12.4983) (45.0071, 12.4192) knots 0 0 0 1 2 2 2
  spline S213 degree 2 poles (45.0071, 12.4192) (44.8935, 12.3377) (44.7872, 12.1352) (44.7872, 11.9746) knots 0 0 0 1 2 2 2
  spline S214 degree 2 poles (44.9305, 10.589) (44.9305, 10.4803) (45.0046, 10.3173) (45.0861, 10.2703) knots 0 0 0 1 2 2 2
  spline S215 degree 2 poles (45.0861, 10.2703) (45.1849, 10.216) (45.4245, 10.1913) (45.6394, 10.1913) knots 0 0 0 1 2 2 2
  line L198 (45.6394, 10.1913) -> (46.0272, 10.1913)
  line L199 (46.0272, 10.1913) -> (46.0272, 11.083)
  line L200 (46.0272, 11.083) -> (45.5678, 11.083)
  spline S216 degree 2 poles (45.5678, 11.083) (45.3776, 11.083) (45.1973, 11.0434) (45.1009, 10.9817) knots 0 0 0 1 2 2 2
  spline S217 degree 2 poles (45.1009, 10.9817) (45.0071, 10.9224) (44.9305, 10.7322) (44.9305, 10.589) knots 0 0 0 1 2 2 2
  line L201 (42.9817, 12.8935) -> (41.9541, 9.8455)
  line L202 (41.9541, 9.8455) -> (41.4552, 9.8455)
  line L203 (41.4552, 9.8455) -> (40.4277, 12.8935)
  line L204 (40.4277, 12.8935) -> (40.855, 12.8935)
  line L205 (40.855, 12.8935) -> (41.1316, 12.0413)
  line L206 (41.1316, 12.0413) -> (42.295, 12.0413)
  line L207 (42.295, 12.0413) -> (42.5716, 12.8935)
  line L208 (42.5716, 12.8935) -> (42.9817, 12.8935)
  line L209 (41.2428, 11.6955) -> (41.7145, 10.2604)
  line L210 (41.7145, 10.2604) -> (42.1838, 11.6955)
  line L211 (42.1838, 11.6955) -> (41.2428, 11.6955)
  spline S218 degree 2 poles (24.6611, 10.1702) (24.6611, 10.3678) (24.8019, 10.7235) (24.9279, 10.847) knots 0 0 0 1 2 2 2
  spline S219 degree 2 poles (24.9279, 10.847) (25.0859, 11.0026) (25.5133, 11.1632) (25.8393, 11.1632) knots 0 0 0 1 2 2 2
  line L212 (25.8393, 11.1632) -> (26.1826, 11.1632)
  line L213 (26.1826, 11.1632) -> (26.1826, 12.2994)
  line L214 (26.1826, 12.2994) -> (26.5877, 12.2994)
  line L215 (26.5877, 12.2994) -> (26.5877, 9.2514)
  line L216 (26.5877, 9.2514) -> (25.822, 9.2514)
  spline S220 degree 2 poles (25.822, 9.2514) (25.5503, 9.2514) (25.1699, 9.3403) (25.0242, 9.4416) knots 0 0 0 1 2 2 2
  spline S221 degree 2 poles (25.0242, 9.4416) (24.8538, 9.5577) (24.6611, 9.9158) (24.6611, 10.1702) knots 0 0 0 1 2 2 2
  spline S222 degree 2 poles (25.0835, 10.1826) (25.0835, 10.0245) (25.1922, 9.7923) (25.3033, 9.7182) knots 0 0 0 1 2 2 2
  spline S223 degree 2 poles (25.3033, 9.7182) (25.3996, 9.654) (25.6565, 9.6021) (25.8467, 9.6021) knots 0 0 0 1 2 2 2
  line L217 (25.8467, 9.6021) -> (26.1826, 9.6021)
  line L218 (26.1826, 9.6021) -> (26.1826, 10.8174)
  line L219 (26.1826, 10.8174) -> (25.906, 10.8174)
  spline S224 degree 2 poles (25.906, 10.8174) (25.659, 10.8174) (25.3552, 10.7383) (25.2564, 10.6346) knots 0 0 0 1 2 2 2
  spline S225 degree 2 poles (25.2564, 10.6346) (25.165, 10.5432) (25.0835, 10.3283) (25.0835, 10.1826) knots 0 0 0 1 2 2 2
  spline S226 degree 2 poles (22.1195, 9.5997) (21.9466, 9.8022) (21.7539, 10.395) (21.7539, 10.7754) knots 0 0 0 1 2 2 2
  spline S227 degree 2 poles (21.7539, 10.7754) (21.7539, 11.1459) (21.9416, 11.7461) (22.1195, 11.9486) knots 0 0 0 1 2 2 2
  spline S228 degree 2 poles (22.1195, 11.9486) (22.3072, 12.1611) (22.8036, 12.3636) (23.1025, 12.3636) knots 0 0 0 1 2 2 2
  spline S229 degree 2 poles (23.1025, 12.3636) (23.4113, 12.3636) (23.9053, 12.1537) (24.0856, 11.9486) knots 0 0 0 1 2 2 2
  spline S230 degree 2 poles (24.0856, 11.9486) (24.261, 11.7461) (24.4487, 11.1508) (24.4487, 10.7754) knots 0 0 0 1 2 2 2
  spline S231 degree 2 poles (24.4487, 10.7754) (24.4487, 10.3925) (24.2585, 9.8096) (24.0831, 9.5997) knots 0 0 0 1 2 2 2
  spline S232 degree 2 poles (24.0831, 9.5997) (23.9053, 9.3971) (23.4088, 9.1872) (23.1025, 9.1872) knots 0 0 0 1 2 2 2
  spline S233 degree 2 poles (23.1025, 9.1872) (22.7913, 9.1872) (22.2924, 9.4045) (22.1195, 9.5997) knots 0 0 0 1 2 2 2
  spline S234 degree 2 poles (22.1763, 10.7754) (22.1763, 10.474) (22.3072, 10.0072) (22.4257, 9.8541) knots 0 0 0 1 2 2 2
  spline S235 degree 2 poles (22.4257, 9.8541) (22.5468, 9.696) (22.8876, 9.5379) (23.1, 9.5379) knots 0 0 0 1 2 2 2
  spline S236 degree 2 poles (23.1, 9.5379) (23.3199, 9.5379) (23.6509, 9.691) (23.7768, 9.8541) knots 0 0 0 1 2 2 2
  spline S237 degree 2 poles (23.7768, 9.8541) (23.8979, 10.0097) (24.0263, 10.479) (24.0263, 10.7754) knots 0 0 0 1 2 2 2
  spline S238 degree 2 poles (24.0263, 10.7754) (24.0263, 11.3756) (23.5224, 12.0129) (23.1, 12.0129) knots 0 0 0 1 2 2 2
  spline S239 degree 2 poles (23.1, 12.0129) (22.6777, 12.0129) (22.1763, 11.3756) (22.1763, 10.7754) knots 0 0 0 1 2 2 2
  line L220 (17.8933, 9.2514) -> (18.659, 12.2994)
  line L221 (18.659, 12.2994) -> (19.1134, 12.2994)
  line L222 (19.1134, 12.2994) -> (19.7334, 9.7701)
  line L223 (19.7334, 9.7701) -> (20.3361, 12.2994)
  line L224 (20.3361, 12.2994) -> (20.7856, 12.2994)
  line L225 (20.7856, 12.2994) -> (21.5637, 9.2514)
  line L226 (21.5637, 9.2514) -> (21.1463, 9.2514)
  line L227 (21.1463, 9.2514) -> (20.5337, 11.7782)
  line L228 (20.5337, 11.7782) -> (19.9261, 9.2514)
  line L229 (19.9261, 9.2514) -> (19.5136, 9.2514)
  line L230 (19.5136, 9.2514) -> (18.901, 11.8078)
  line L231 (18.901, 11.8078) -> (18.2909, 9.2514)
  line L232 (18.2909, 9.2514) -> (17.8933, 9.2514)
  line L233 (17.5302, 12.2994) -> (17.5302, 9.2514)
  line L234 (17.5302, 9.2514) -> (15.6233, 9.2514)
  line L235 (15.6233, 9.2514) -> (15.6233, 9.612)
  line L236 (15.6233, 9.612) -> (17.1251, 9.612)
  line L237 (17.1251, 9.612) -> (17.1251, 10.4469)
  line L238 (17.1251, 10.4469) -> (15.7246, 10.4469)
  line L239 (15.7246, 10.4469) -> (15.7246, 10.8075)
  line L240 (15.7246, 10.8075) -> (17.1251, 10.8075)
  line L241 (17.1251, 10.8075) -> (17.1251, 11.9388)
  line L242 (17.1251, 11.9388) -> (15.6233, 11.9388)
  line L243 (15.6233, 11.9388) -> (15.6233, 12.2994)
  line L244 (15.6233, 12.2994) -> (17.5302, 12.2994)
  line L245 (12.8198, 12.2994) -> (13.346, 12.2994)
  line L246 (13.346, 12.2994) -> (14.3093, 11.0866)
  line L247 (14.3093, 11.0866) -> (14.7736, 11.0866)
  line L248 (14.7736, 11.0866) -> (14.7736, 12.2994)
  line L249 (14.7736, 12.2994) -> (15.1787, 12.2994)
  line L250 (15.1787, 12.2994) -> (15.1787, 9.2514)
  line L251 (15.1787, 9.2514) -> (14.3932, 9.2514)
  spline S240 degree 2 poles (14.3932, 9.2514) (14.1314, 9.2514) (13.7782, 9.3082) (13.6177, 9.4119) knots 0 0 0 1 2 2 2
  spline S241 degree 2 poles (13.6177, 9.4119) (13.4571, 9.5157) (13.2719, 9.8392) (13.2719, 10.0788) knots 0 0 0 1 2 2 2
  spline S242 degree 2 poles (13.2719, 10.0788) (13.2719, 10.4123) (13.6127, 10.8643) (13.9042, 10.973) knots 0 0 0 1 2 2 2
  line L252 (13.9042, 10.973) -> (12.8198, 12.2994)
  spline S243 degree 2 poles (13.6942, 10.1109) (13.6942, 9.9776) (13.7881, 9.7726) (13.8869, 9.7059) knots 0 0 0 1 2 2 2
  spline S244 degree 2 poles (13.8869, 9.7059) (13.9733, 9.6491) (14.203, 9.6021) (14.371, 9.6021) knots 0 0 0 1 2 2 2
  line L253 (14.371, 9.6021) -> (14.7736, 9.6021)
  line L254 (14.7736, 9.6021) -> (14.7736, 10.7482)
  line L255 (14.7736, 10.7482) -> (14.4179, 10.7482)
  spline S245 degree 2 poles (14.4179, 10.7482) (14.2426, 10.7482) (13.9635, 10.6865) (13.8671, 10.5901) knots 0 0 0 1 2 2 2
  spline S246 degree 2 poles (13.8671, 10.5901) (13.7782, 10.5062) (13.6942, 10.269) (13.6942, 10.1109) knots 0 0 0 1 2 2 2
  point P0 (70, 32)
  constraints: 6 other
emboss "Emboss1" sketch "Sketch5" operation cut depth 0.5 direction (0, -1, 0)
sketch "Sketch6" plane through (0, 0, 3) normal (0, 0, 1) x (1, 0, 0)
  line L0 (80, 53.5) -> (-80, 53.5) projected
  line L1 (-80, 53.5) -> (-80, -53.5) projected
  line L2 (-80, -53.5) -> (80, -53.5) projected
  line L3 (80, -53.5) -> (80, 53.5) projected
  line L4 (70, -43.5) -> (70, 43.5) projected
  line L5 (-70, -43.5) -> (70, -43.5) projected
  line L6 (-70, 43.5) -> (-70, -43.5) projected
  line L7 (70, 43.5) -> (-70, 43.5) projected
  line L8 (-80, 53.5) -> (-80, -53.5) construction
  line L9 (80, 53.5) -> (-80, -53.5) construction
  line L10 (-80, -53.5) -> (-80, 53.5) construction
  line L11 (-80, 53.5) -> (80, -53.5) construction
  line L12 (80, 0) -> (-80, 0) construction
  line L13 (80, 53.5) -> (-80, 53.5) construction
  line L14 (0, 53.5) -> (0, -53.5) construction
  line L15 (-80, -53.5) -> (-70, -43.5) construction
  line L16 (70, 43.5) -> (80, 53.5) construction
  line L17 (-68, -41.5) -> (-68, 41.5) construction
  line L18 (67.8241, 41.3241) -> (-68, -41.5) construction
  line L19 (-68, -41.5) -> (-70, 43.5) construction
  line L20 (-70, 43.5) -> (-80, 53.5) construction
  line L21 (70, -43.5) -> (80, -53.5) construction
  line L22 (68, -41.5) -> (-68, 41.5) construction
  circle A0 centre (75, -48.5) radius 2
  circle A1 centre (-75, -48.5) radius 2
  circle A2 centre (75, 48.5) radius 2
  circle A3 centre (-75, 48.5) radius 2
  point P0 (0, 0)
  dimension "d18" = 4
  constraints: 24 end point, 5 midpoint, 4 centre point, 3 equal length, 3 symmetric about line, 2 point on line, 1 perpendicular, 3 other
  measures "d18" diameter of A0
extrude "Extrusion5" cut sketch "Sketch6" against normal blind 25.4 contours A0 | A1 | A2 | A3
fillet "Fillet1" radius 1.7 4 edges at (0, 43.5, 32) (70, 0, 32) (0, -43.5, 32) (-70, 0, 32)
chamfer "Chamfer1" distance 0.7 angle 45 4 edges at (73, 48.5, 3) (-77, 48.5, 3) (-77, -48.5, 3) (73, -48.5, 3)
fillet "Fillet2" radius 1 4 edges at (-70, 0, 3) (0, 43.5, 3) (70, 0, 3) (0, -43.5, 3)
